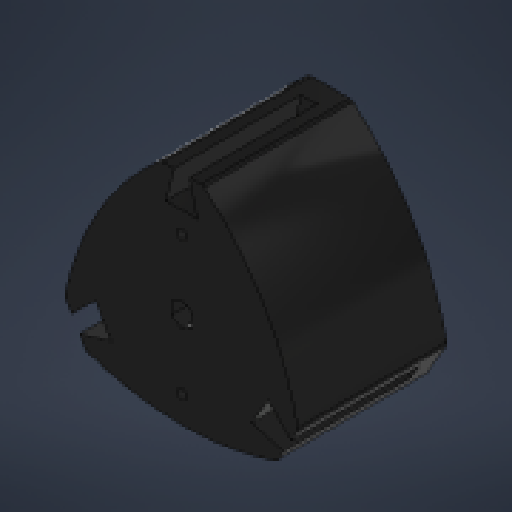
# Autodesk Inventor part: 3DPRINT,HUB
Saved by Autodesk Inventor 2026.1 (Build 301233020, 233B)
## iProperties
Created: 2026-02-05
Part Number: 3DPRINT,HUB
Material: ABS Plastic
Document SubType Name: Modeling
Designer: Owen L
Density: 0.316929 g/cm^3
Appearance: Smooth - Black
Mass: 362.874 g
Surface Area: 937.42 cm^2
Volume: 1144.97 cm^3
Author: Owen L
Autodesk Inventor part; units mm, degrees
ref_plane "XZ Plane" through (0, 0, 0) normal (0, 1, 0) x (-1, 0, 0)
ref_plane "XY Plane" through (0, 0, 0) normal (0, 0, 1) x (1, 0, 0)
sketch "Sketch1" plane through (0, 0, 0) normal (0, 0, 1) x (1, 0, 0)
  line L0 (0, 0) -> (0, 50.8) construction
  line L1 (-12.7, 50.8) -> (12.7, 50.8)
  line L2 (-37.6441, -36.3985) -> (-50.3441, -14.4015)
  line L3 (50.3441, -14.4015) -> (37.6441, -36.3985)
  arc A0 (-12.7, 50.8) -> (-50.3441, -14.4015) centre (113.3348, -65.4339) ccw
  arc A1 (50.3441, -14.4015) -> (12.7, 50.8) centre (-113.3348, -65.4339) ccw
  arc A2 (-37.6441, -36.3985) -> (37.6441, -36.3985) centre (0, 130.8678) ccw
  dimension "d0" = 50.8
  dimension "d1" = 25.4
  dimension "d4" = 360
  dimension "d149" = 171.45
  constraints: 8 end point, 6 point on circle, 3 centre point, 2 equal radius, 1 horizontal, 1 midpoint, 1 vertical, 10 other
  measures "d0" distance of L0.start L0.end
  measures "d1" distance of L1.start L1.end
  measures "d149" radius of A0
extrude "Extrusion5" add sketch "Sketch1" along normal mid plane 88.9
ref_plane "Work Plane5" through (0, 0, 44.45) normal (0, 0, 1) x (1, 0, 0)
sketch "Sketch7" plane through (0, 0, 44.45) normal (0, 0, 1) x (1, 0, 0)
  line L0 (12.7, 50.8) -> (-12.7, 50.8) projected
  line L1 (0, 0) -> (0, 50.8) construction
  line L2 (-5.08, 50.8) -> (-10.795, 31.75)
  line L3 (-10.795, 31.75) -> (10.795, 31.75)
  line L4 (10.795, 31.75) -> (5.08, 50.8)
  dimension "d122" = 21.59
  dimension "d147" = 10.16
  dimension "d148" = 19.05
  constraints: 8 end point, 2 point on line, 1 equal length, 1 midpoint, 1 other
  measures "d122" distance of L2.end L3.end
  measures "d147" distance of L2.start L4.end
  measures "d148" distance between parallel lines of L3 L0
extrude "Extrusion6" cut sketch "Sketch7" against normal blind 76.2
pattern_circular "Circular Pattern3" count 3 over 360 about axis through (0, 0, -10) along (0, 0, 1) of "Extrusion6"
fillet "Fillet3" radius 3.175 6 edges at (-37.6441, -36.3985, 0) (-50.3441, -14.4015, 0) (-12.7, 50.8, 0) (37.6441, -36.3985, 0) (50.3441, -14.4015, 0) (12.7, 50.8, 0)
sketch "Sketch9" plane through (0, 0, -44.45) normal (0, 0, -1) x (-1, 0, 0)
  point P0 (0, 0)
  point P1 (0, -44.45)
  point P2 (38.4948, -22.225)
  point P3 (38.4948, 22.225)
  point P4 (0, 44.45)
  point P5 (-38.4948, 22.225)
  point P6 (-38.4948, -22.225)
  dimension "d93" = 44.45
  dimension "d96" = 360
  constraints: 1 vertical alignment, 7 other
  measures "d93" distance of point (0, 0) point (0, -44.45)
hole "Hole1" at (-38.4948, -22.225, -44.45) at (0, 44.45, -44.45) at (38.4948, -22.225, -44.45) direction (0, 0, 1) diameter 6.12 depth 12.7 tip angle 118
sketch "Sketch10" plane through (0, 0, 44.45) normal (0, 0, 1) x (1, 0, 0)
  point P0 (0, 0)
  point P1 (0, -25.4)
  point P2 (21.997, 12.7)
  point P3 (-21.997, 12.7)
  dimension "d107" = 360
  dimension "d109" = 25.4
  constraints: 1 vertical alignment, 4 other
  measures "d109" distance of point (0, -25.4) point (0, 0)
hole "Hole2" at (0, -25.4, 44.45) at (21.997, 12.7, 44.45) at (-21.997, 12.7, 44.45) direction (0, 0, -1) diameter 6.12 depth 12.7 tip angle 118
sketch "Sketch11" plane through (0, 0, -44.45) normal (0, 0, -1) x (-1, 0, 0)
  line L0 (-6.4135, -3.7028) -> (-6.4135, 3.7028)
  line L1 (-6.4135, 3.7028) -> (0, 7.4057)
  line L2 (0, 7.4057) -> (6.4135, 3.7028)
  line L3 (6.4135, 3.7028) -> (6.4135, -3.7028)
  line L4 (6.4135, -3.7028) -> (0, -7.4057)
  line L5 (0, -7.4057) -> (-6.4135, -3.7028)
  point P0 (0, 0)
  point P1 (0, 0)
  dimension "d118" = 12.827
  constraints: 12 end point, 1 coincident, 1 vertical, 13 other
  measures "d118" distance between parallel lines of L3 L0
extrude "Extrusion8" cut sketch "Sketch11" against normal through all
ref_plane "Work Plane6" through (38.1, 0, 0) normal (1, 0, 0) x (0, 1, 0)
ref_plane "Work Plane7" through (-38.1, 0, 0) normal (1, 0, 0) x (0, 1, 0)
body "Solid3"
